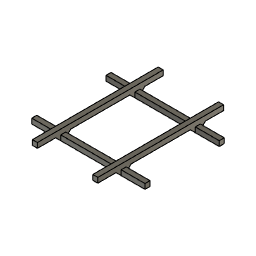
底架（仿） v1 (Autodesk Fusion 360 design; units mm, degrees)
Autodesk Fusion 360 part; units mm, degrees
sketch "草图1" plane through (0, 0, 0) normal (0, 0, 1) x (1, 0, 0)
  line L0 (110, -137.5) -> (-110, -137.5)
  line L1 (-110, -137.5) -> (-110, 137.5)
  line L2 (-110, 137.5) -> (110, 137.5)
  line L3 (110, 137.5) -> (110, -137.5)
  line L4 (110, -137.5) -> (-110, 137.5) construction
  line L5 (-110, -137.5) -> (110, 137.5) construction
  line L6 (130, -157.5) -> (-130, -157.5)
  line L7 (-130, -157.5) -> (-130, 157.5)
  line L8 (-130, 157.5) -> (130, 157.5)
  line L9 (130, 157.5) -> (130, -157.5)
  line L10 (130, -157.5) -> (-130, 157.5) construction
  line L11 (-130, -157.5) -> (130, 157.5) construction
  line L12 (110, 137.5) -> (225, 137.5)
  line L13 (225, 137.5) -> (-225, 137.5)
  line L14 (0, 0) -> (0, 157.5) construction
  line L15 (0, 0) -> (0, -157.5) construction
  line L16 (-110, 137.5) -> (-110, 250)
  line L17 (-110, 250) -> (-110, -250)
  line L18 (0, 0) -> (-130, 0) construction
  line L19 (-225, 250) -> (225, 250)
  line L20 (225, 250) -> (225, -250)
  line L21 (225, -250) -> (-225, -250)
  line L22 (-225, -250) -> (-225, 250)
  line L23 (-225, 250) -> (225, -250) construction
  line L24 (225, 250) -> (-225, -250) construction
  line L25 (-130, 250) -> (-130, -250)
  line L26 (225, -157.5) -> (-225, -157.5)
  line L27 (-225, -137.5) -> (225, -137.5)
  line L28 (110, 250) -> (110, -250)
  line L29 (130, -250) -> (130, 250)
  line L30 (225, 157.5) -> (-225, 157.5)
  point P0 (-110, 0)
  dimension "d1" = 220
  dimension "d2" = 275
  dimension "d3" = 20
  dimension "d4" = 20
  dimension "d5" = 450
  dimension "d6" = 95
  dimension "d7" = 95
  dimension "d8" = 500
  dimension "d9" = 92.5
  constraint horizontal L0
  constraint perpendicular L0 L1
  constraint parallel L0 L2
  constraint parallel L1 L3
  constraint coincident L4 L14.start
  constraint coincident L5 L14.start
  constraint coincident L14.start L15.start
  constraint horizontal L6
  constraint perpendicular L6 L7
  constraint parallel L6 L8
  constraint parallel L7 L9
  constraint coincident L10 L14.start
  constraint coincident L11 L14.start
  constraint perpendicular L3 L12
  constraint perpendicular L7 L13
  constraint midpoint L8 L14.end
  constraint midpoint L6 L15.end
  constraint symmetric L12.end L13.end L14
  constraint perpendicular L13 L16
  constraint perpendicular L6 L17
  constraint midpoint L7 L18.end
  constraint coincident L18 P0
  constraint symmetric L16.end L17.end L18
  constraint horizontal L19
  constraint perpendicular L19 L20
  constraint parallel L19 L21
  constraint parallel L20 L22
  constraint coincident L23 L14.start
  constraint coincident L24 L14.start
  constraint coincident L13.end L22
  constraint coincident L16.end L19
  constraint coincident L19 L25.start
  constraint coincident L21 L25.end
  constraint perpendicular L21 L25
  constraint coincident L20 L26.start
  constraint coincident L22 L26.end
  constraint perpendicular L22 L26
  constraint coincident L22 L27.start
  constraint coincident L20 L27.end
  constraint perpendicular L20 L27
  constraint coincident L19 L28.start
  constraint coincident L21 L28.end
  constraint perpendicular L21 L28
  constraint coincident L21 L29.start
  constraint coincident L19 L29.end
  constraint perpendicular L19 L29
  constraint coincident L20 L30.start
  constraint coincident L22 L30.end
  constraint perpendicular L22 L30
  measures "d1" distance of L1.end L2.end
  measures "d2" distance of L0.end L1.end
  measures "d3" distance of L3 L9
  measures "d4" distance of L2 L8
  measures "d5" distance of L12.end L13.end
  measures "d6" distance of L9 L12.end
  measures "d7" distance of L7 L13.end
  measures "d8" distance of L16.end L17.end
  measures "d9" distance of L8 L16.end
extrude "拉伸1" add sketch "草图1" along normal blind 20 contours L3 L9 L12 L13 L27 L28 L29 | L6 L9 L26 L27 L28 L29 | L1 L7 L13 L17 L25 L27 | L6 L7 L17 L25 L26 L27 | L8 L9 L12 L13 L28 L29 L30 | L6 L21 L26 L28 L29 | L7 L8 L13 L16 L17 L25 L30 | L6 L17 L21 L25 L26 | L8 L19 L28 L29 L30 | L8 L16 L17 L19 L25 L30 makes body 1 at (-110, 83.3333, 6.6667) makes body 2 at (130, 83.3333, 6.6667)
extrude "拉伸2" add sketch "草图1" against normal blind 20 contours L0 L6 L17 L26 L27 L28 | L6 L9 L26 L27 L28 L29 | L6 L7 L17 L25 L26 L27 | L8 L9 L12 L13 L28 L29 L30 | L2 L8 L13 L16 L17 L28 L30 | L9 L20 L26 L27 L29 | L7 L8 L13 L16 L17 L25 L30 | L7 L22 L25 L26 L27 | L9 L12 L13 L20 L29 L30 | L7 L13 L22 L25 L30 bodies 1 2
chamfer "倒角1" distance 20 angle 45 8 edges at (-120, -157.5, 0) (120, -157.5, 0) (-120, 137.5, 0) (120, 137.5, 0) (-120, -137.5, 0) (-120, 157.5, 0) (120, 157.5, 0) (120, -137.5, 0) on bodies 1
